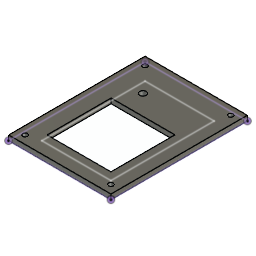
HackPad Top piece (Autodesk Fusion 360 design; units mm, degrees)
part number: 2026-02-17-20-08-38-436
Autodesk Fusion 360 part; units mm, degrees
sketch "Sketch1" plane through (0, 0, 0) normal (0, 0, 1) x (1, 0, 0)
  line L0 (0, 0) -> (61.5, 0)
  line L1 (61.5, 0) -> (61.5, 82)
  line L2 (61.5, 82) -> (0, 82)
  line L3 (0, 82) -> (0, 0)
  dimension "d1" = 82
  dimension "d2" = 61.5
  constraint horizontal L0
  constraint vertical L1
  constraint horizontal L2
  constraint vertical L3
  constraint coincident L0.start L3.end
  measures "d1" distance of L0.start L2.end
  measures "d2" distance of L0.start L0.end
extrude "Extrude1" add sketch "Sketch1" along normal blind 3
sketch "Sketch2" plane through (0, 0, 3) normal (0, 0, 1) x (-1, 0, 0)
  line L0 (0, -82) -> (0, 0)
  line L1 (0, 0) -> (-61.5, 0)
  line L2 (-61.5, 0) -> (-61.5, -82)
  line L3 (-61.5, -82) -> (0, -82)
  circle A0 centre (-5, -5) radius 1.45
  circle A1 centre (-5, -77) radius 1.45
  circle A2 centre (-56.5, -77) radius 1.45
  circle A3 centre (-56.5, -5) radius 1.45
  dimension "d5" = 2.9
  dimension "d6" = 5
  dimension "d7" = 5
  dimension "d8" = 2.9
  dimension "d9" = 5
  dimension "d10" = 5
  dimension "d11" = 2.9
  dimension "d12" = 5
  dimension "d13" = 5
  dimension "d14" = 2.9
  dimension "d15" = 5
  dimension "d16" = 5
  measures "d5" diameter of A0
  measures "d6" distance of L0 A0.centre
  measures "d7" distance of L1 A0.centre
  measures "d8" diameter of A1
  measures "d9" distance of L3 A1.centre
  measures "d10" distance of L0 A1.centre
  measures "d11" diameter of A2
  measures "d12" distance of L3 A2.centre
  measures "d13" distance of L2 A2.centre
  measures "d14" diameter of A3
  measures "d15" distance of L2 A3.centre
  measures "d16" distance of L1 A3.centre
extrude "Extrude2" cut sketch "Sketch2" against normal blind 3 contours A0 | A1 | A2 | A3
sketch "Sketch3" plane through (0, 0, 0) normal (0, 0, 1) x (1, 0, 0)
  line L0 (10, 72) -> (51.5, 72)
  line L1 (51.5, 72) -> (51.5, 10)
  line L2 (51.5, 10) -> (10, 10)
  line L3 (10, 10) -> (10, 72)
  line L4 (61.5, 82) -> (0, 82)
  line L5 (61.5, 0) -> (61.5, 82)
  line L6 (0, 0) -> (61.5, 0)
  line L7 (0, 82) -> (0, 0)
  dimension "d19" = 10
  dimension "d20" = 10
  dimension "d21" = 10
  dimension "d22" = 10
  constraint horizontal L0
  constraint vertical L1
  constraint horizontal L2
  constraint vertical L3
  measures "d19" distance of L0 L4
  measures "d20" distance of L1 L5
  measures "d21" distance of L2 L6
  measures "d22" distance of L3 L7
sketch "Sketch4" plane through (0, 0, 0) normal (0, 0, 1) x (1, 0, 0)
sketch "Sketch5" plane through (0, 0, 0) normal (0, 0, 1) x (1, 0, 0)
sketch "Sketch6" plane through (0, 0, 0) normal (0, 0, 1) x (1, 0, 0)
  line L0 (49.9, 50) -> (11.6, 50)
  line L1 (11.6, 50) -> (11.6, 11.6)
  line L2 (11.6, 11.6) -> (49.9, 11.6)
  line L3 (49.9, 11.6) -> (49.9, 50)
  line L4 (51.5, 72) -> (51.5, 10)
  line L5 (10, 10) -> (10, 72)
  line L6 (51.5, 10) -> (10, 10)
  line L7 (10, 72) -> (51.5, 72)
  dimension "d23" = 1.6
  dimension "d24" = 1.6
  dimension "d25" = 1.6
  dimension "d26" = 22
  constraint horizontal L0
  constraint vertical L1
  constraint horizontal L2
  constraint vertical L3
  measures "d23" distance of L3 L4
  measures "d24" distance of L1 L5
  measures "d25" distance of L2 L6
  measures "d26" distance of L0 L7
sketch "Sketch7" plane through (0, 0, 0) normal (0, 0, 1) x (1, 0, 0)
  circle A0 centre (18.7, 62) radius 2
  line L0 (10, 72) -> (51.5, 72)
  line L1 (10, 10) -> (10, 72)
  dimension "d30" = 4
  dimension "d31" = 10
  dimension "d32" = 8.7
  measures "d30" diameter of A0
  measures "d31" distance of A0.centre L0
  measures "d32" distance of A0.centre L1
extrude "Extrude3" cut sketch "Sketch6" sketch "Sketch7" along normal blind 3 contours L0 L1 L2 L3 of sketch 2
